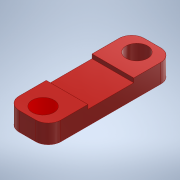
# Autodesk Inventor part: LED_Strip_Halter_einzeln
Saved by Autodesk Inventor 2021.2 (Build 252289000, 289)
## iProperties
Part Number: LED_Strip_Halter_einzeln
Material: PA 6 schwarz
Document SubType Name: Modeling
Designer: SRORF
Mass: 2.02202 g
Surface Area: 13.2849 cm^2
Volume: 1.7737 cm^3
Density: 1.14 g/cm^3
Appearance: Orangerot
ROT_Density: 1.0
PDB_Ident_Ver: =<PDB_Ident> <PDB_Version>
ROT_Weight: 0.002 kg
ROT_Weight_Num: 0.0020220180089347735
Author: SRORF
Autodesk Inventor part; units mm, degrees
ref_plane "YZ Plane" through (0, 0, 0) normal (1, 0, 0) x (0, 1, 0)
ref_plane "XZ Plane" through (0, 0, 0) normal (0, 1, 0) x (-1, 0, 0)
ref_plane "XY Plane" through (0, 0, 0) normal (0, 0, 1) x (1, 0, 0)
sketch "Skizze2" plane through (0, 0, 0) normal (0, 0, 1) x (1, 0, 0)
  line L0 (-5, 7) -> (5, 7)
  line L1 (5, 7) -> (5, -7)
  line L2 (5, -7) -> (-5, -7)
  line L3 (-5, -7) -> (-5, 7)
  line L4 (0, 9.8) -> (0, -9.8) projected
  line L5 (-7, 0) -> (7, 0) projected
  point P0 (0, 0)
  point P1 (-5, 0)
  point P2 (0, 7)
  dimension "d0" = 14
  dimension "d1" = 10
  constraints: 8 end point, 2 midpoint, 2 parallel, 2 point on line, 1 horizontal, 1 perpendicular
  measures "d0" distance of L2.end L0.start
  measures "d1" distance of L0.start L0.end
extrude "Extrusion1" add sketch "Skizze2" along normal blind 3.5
sketch "Skizze3" plane through (0, 0, 3.5) normal (0, 0, 1) x (1, 0, 0)
  line L0 (5, -7) -> (5, 7) projected
  line L1 (5, 7) -> (-5, 7) projected
  line L2 (-5, 7) -> (-5, -7) projected
  line L3 (-5, -7) -> (5, -7) projected
  line L4 (5, 7) -> (-5, 7)
  line L5 (-5, 7) -> (-5, 5.5)
  line L6 (-5, 5.5) -> (5, 5.5)
  line L7 (5, 5.5) -> (5, 7)
  line L8 (-5, 7) -> (-5, -7) projected
  line L9 (-5, -7) -> (5, -7)
  line L10 (5, -7) -> (5, -5.5)
  line L11 (5, -5.5) -> (-5, -5.5)
  line L12 (-5, -5.5) -> (-5, -7)
  point P0 (0, 0)
  dimension "d4" = 1.5
  dimension "d5" = 1.5
  constraints: 16 end point, 4 parallel, 2 horizontal, 2 perpendicular, 2 point on line
  measures "d4" distance between parallel lines of L3 L11
  measures "d5" distance between parallel lines of L1 L6
extrude "Extrusion2" add sketch "Skizze3" along normal blind 1 contours L3 L2 L11 L0 | L6 L2 L1 L0
sketch "Skizze4" plane through (0, 0, 0) normal (0, 0, -1) x (-1, 0, 0)
  line L0 (5, -7) -> (-5, -7) projected
  line L1 (5, -7) -> (-5, -7)
  line L2 (-5, -7) -> (-5, -15)
  line L3 (-5, -15) -> (5, -15)
  line L4 (5, -15) -> (5, -7)
  line L5 (-5, 7) -> (5, 7)
  line L6 (5, 7) -> (5, 15)
  line L7 (5, 15) -> (-5, 15)
  line L8 (-5, 15) -> (-5, 7)
  line L9 (5, -7) -> (-5, -7) projected
  line L10 (-5, 7) -> (5, 7) projected
  line L11 (5, 7) -> (5, -7) projected
  line L12 (-5, -7) -> (-5, 7) projected
  line L13 (5, 5.5) -> (5, -5.5) projected
  point P0 (0, 0)
  point P1 (-5, -7)
  point P2 (0, -15)
  point P3 (0, -11)
  point P4 (0, 11)
  point P5 (5, -11)
  point P6 (5, 11)
  dimension "d8" = 8
  dimension "d9" = 8
  dimension "d31" = 10
  dimension "d32" = 22
  constraints: 16 end point, 4 parallel, 4 point on line, 3 midpoint, 2 horizontal, 2 horizontal alignment, 2 perpendicular, 2 vertical alignment, 1 collinear
  measures "d8" distance between parallel lines of L0 L3
  measures "d9" distance of L7.end L5.start
  measures "d31" distance of L2.end L3.end
  measures "d32" distance of point (0, -11) point (0, 11)
extrude "Extrusion3" add sketch "Skizze4" against normal up to surface (4.5 mm away) contours L4 L3 L2 L0 | L8 L7 L6 L5
sketch "Skizze5" plane through (0, 0, 0) normal (0, 0, -1) x (-1, 0, 0)
  line L0 (-5, 5.5) -> (-5, 15) projected
  line L1 (-5, -5.5) -> (-5, -15) projected
  line L2 (-5, -15) -> (5, -15) projected
  line L3 (5, 15) -> (-5, 15) projected
  line L4 (-7, 0) -> (7, 0) projected
  point P0 (0, 11.25)
  point P1 (0, -11.25)
  point P2 (0, -15)
  point P3 (0, 15)
  dimension "d39" = 22.5
  dimension "d40" = 11.25
  constraints: 2 midpoint, 2 vertical alignment
  measures "d39" distance of point (0, -11.25) point (0, 11.25)
  measures "d40" distance from line of L4 point (0, -11.25)
hole "Bohrung1" at (0, -11.25, 0) direction (0, 0, 1) diameter 5.2 end through all
fillet "Rundung1" radius 3 4 edges at (-5, -15, 2.25) (5, -15, 2.25) (5, 15, 2.25) (-5, 15, 2.25)
pattern_linear "Rechteckige Anordnung1" count 2 spacing 22.5 along (0, 1, 0) of "Bohrung1"
equation "\"d5\" = d4"
equation "\"d9\" = d8"
equation "\"d24\" = d34"
equation "\"d34\" = 22.5"
